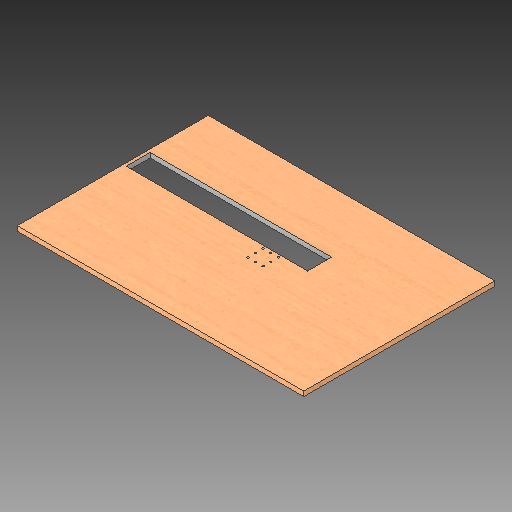
# Autodesk Inventor part: face-lateral
Saved by Autodesk Inventor 2017 (Build 210142000, 142)
## iProperties
Created: 2018-04-02
Part Number: face-lateral
Material: Generic
Document SubType Name: Modeling
Designer: franc
Density: 1 g/cm^3
Appearance: Default
Author: franc
Autodesk Inventor part; units mm, degrees
ref_plane "YZ Plane" through (0, 0, 0) normal (1, 0, 0) x (0, 1, 0)
ref_plane "XZ Plane" through (0, 0, 0) normal (0, 1, 0) x (-1, 0, 0)
ref_plane "XY Plane" through (0, 0, 0) normal (0, 0, 1) x (1, 0, 0)
sketch "Esquisse1" plane through (0, 0, 0) normal (0, 1, 0) x (-1, 0, 0)
  line L0 (98.2051, 94.359) -> (-201.7949, 94.359)
  line L1 (-201.7949, 94.359) -> (-201.7949, -105.641)
  line L2 (-201.7949, -105.641) -> (98.2051, -105.641)
  line L3 (98.2051, -105.641) -> (98.2051, 94.359)
  point P0 (0, 0)
  dimension "d0" = 200
  dimension "d1" = 300
  constraints: 8 end point, 2 parallel, 1 horizontal, 1 perpendicular
  measures "d0" distance of L2.end L0.start
  measures "d1" distance of L1.end L2.end
extrude "Extrusion1" add sketch "Esquisse1" along normal blind 5
sketch "Esquisse2" plane through (0, 5, 0) normal (0, 1, 0) x (1, 0, 0)
  line L0 (84.9258, 26.641) -> (-85.0623, 26.641) projected
  line L1 (84.9258, 31.641) -> (-85.0623, 31.641) projected
  line L2 (-85.0623, 26.641) -> (-85.0623, 31.641) projected
  line L3 (84.9258, 26.641) -> (84.9258, 31.641) projected
  line L4 (-95.0623, 16.641) -> (94.9258, 16.641)
  line L5 (94.9258, 16.641) -> (94.9258, 41.641)
  line L6 (94.9258, 41.641) -> (-95.0623, 41.641)
  line L7 (-95.0623, 41.641) -> (-95.0623, 16.641)
  point P0 (0, 0)
  dimension "d4" = 10
  dimension "d5" = 10
  dimension "d6" = 10
  dimension "d7" = 10
  constraints: 8 end point, 2 parallel, 1 horizontal, 1 perpendicular
  measures "d4" distance between parallel lines of L4 L0
  measures "d5" distance between parallel lines of L6 L1
  measures "d6" distance between parallel lines of L7 L2
  measures "d7" distance between parallel lines of L3 L5
extrude "Extrusion2" cut sketch "Esquisse2" against normal through all contours L0 L2 L1 L3 | L7 L6 L5 L4
sketch "Esquisse3" plane through (0, 0, 0) normal (0, -1, 0) x (1, 0, 0)
  line L0 (71.7949, -22.641) -> (62.7949, -22.641) projected
  line L1 (71.7949, 11.359) -> (71.7949, -22.641) projected
  line L2 (71.7949, 11.359) -> (62.7949, 11.359) projected
  line L3 (62.7949, 10.359) -> (62.7949, 11.359) projected
  line L4 (62.7949, 10.359) -> (54.7949, 10.359) projected
  line L5 (54.7949, 10.359) -> (54.7949, 11.359) projected
  line L6 (54.7949, 11.359) -> (46.7949, 11.359) projected
  line L7 (46.7949, -22.641) -> (46.7949, 11.359) projected
  line L8 (54.7949, -22.641) -> (46.7949, -22.641) projected
  line L9 (54.7949, -21.641) -> (54.7949, -22.641) projected
  line L10 (62.7949, -21.641) -> (54.7949, -21.641) projected
  line L11 (62.7949, -21.641) -> (62.7949, -22.641) projected
  circle A0 centre (67.2949, -5.641) radius 1 projected
  circle A1 centre (67.2949, -13.641) radius 1 projected
  circle A2 centre (67.2949, 2.359) radius 1 projected
  circle A3 centre (59.2949, 2.359) radius 1 projected
  circle A4 centre (51.2949, -5.641) radius 1 projected
  circle A5 centre (51.2949, -13.641) radius 1 projected
  circle A6 centre (51.2949, 2.359) radius 1 projected
  circle A7 centre (59.2949, -13.641) radius 1 projected
  arc A8 (56.2949, -2.9953) -> (56.2949, -8.2868) centre (59.2949, -5.641) ccw projected
  line L12 (56.2949, -2.9953) -> (56.2949, -0.641) projected
  line L13 (56.2949, -0.641) -> (62.2949, -0.641) projected
  line L14 (62.2949, -0.641) -> (62.2949, -2.9953) projected
  arc A9 (62.2949, -8.2868) -> (62.2949, -2.9953) centre (59.2949, -5.641) ccw projected
  line L15 (62.2949, -8.2868) -> (62.2949, -10.641) projected
  line L16 (62.2949, -10.641) -> (56.2949, -10.641) projected
  line L17 (56.2949, -10.641) -> (56.2949, -8.2868) projected
  point P0 (0, 0)
extrude "Extrusion3" cut sketch "Esquisse3" against normal through all contours A0 | A1 | A2 | A3 | A4 | A5 | A6 | A7
